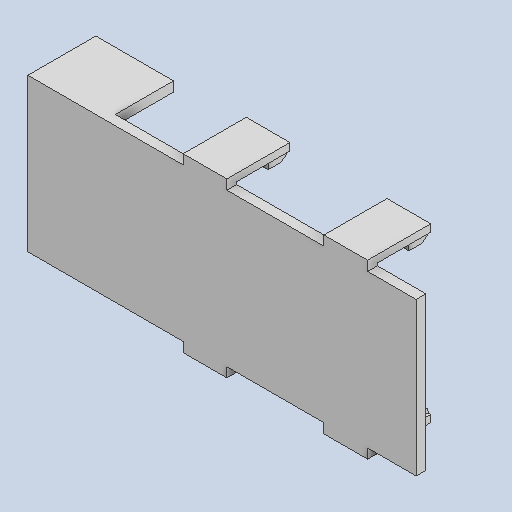
# Autodesk Inventor part: np2_cap_open_top
Saved by Autodesk Inventor 2025 (Build 290162000, 162)
## iProperties
Created: 2023-11-21
Part Number: np2_cap_open_top
Material: Generic
Document SubType Name: Modeling
Designer: mmelin
Density: 1 g/cm^3
Appearance: Default
Author: mmelin
Autodesk Inventor part; units mm, degrees
ref_plane "YZ Plane" through (0, 0, 0) normal (1, 0, 0) x (0, 1, 0)
ref_plane "XZ Plane" through (0, 0, 0) normal (0, 1, 0) x (-1, 0, 0)
sketch "Sketch1" plane through (0, 0, 0) normal (0, 0, 1) x (1, 0, 0)
  line L0 (1, -0.6) -> (1, -5.45) projected
  line L1 (-15, 0) -> (-11.6, 0)
  line L2 (-6.8, -6.3) -> (-8.6, -6.3) projected
  line L3 (-8.6, 0) -> (-6.8, 0) projected
  line L4 (-2.8, 0) -> (-1, 0) projected
  line L5 (-6.8, -6.3) -> (-8.6, -6.3) projected
  line L6 (-1, -6.3) -> (-2.8, -6.3) projected
  line L7 (-8.6, -6.3) -> (-6.8, -6.3)
  line L8 (-6.8, -6.3) -> (-6.8, -6.7)
  line L9 (-6.8, -6.7) -> (-8.6, -6.7)
  line L10 (-8.6, -6.7) -> (-8.6, -6.3)
  line L11 (-8.6, 0) -> (-6.8, 0)
  line L12 (-6.8, 0) -> (-6.8, 0.4)
  line L13 (-6.8, 0.4) -> (-8.6, 0.4)
  line L14 (-8.6, 0.4) -> (-8.6, 0)
  line L15 (-2.8, 0) -> (-1, 0)
  line L16 (-1, 0) -> (-1, 0.4)
  line L17 (-1, 0.4) -> (-2.8, 0.4)
  line L18 (-2.8, 0.4) -> (-2.8, 0)
  line L19 (-2.8, -6.3) -> (-1, -6.3)
  line L20 (-1, -6.3) -> (-1, -6.7)
  line L21 (-1, -6.7) -> (-2.8, -6.7)
  line L22 (-2.8, -6.7) -> (-2.8, -6.3)
  line L23 (-8.6, -5.9) -> (-8.6, -6.3) projected
  line L24 (-6.8, -5.9) -> (-6.8, -6.3) projected
  line L25 (-2.8, -5.9) -> (-2.8, -6.3) projected
  line L26 (-1, -5.9) -> (-1, -6.3) projected
  line L27 (1, -6.3) -> (-15, -6.3)
  line L28 (-15, -6.3) -> (-15, 0)
  line L29 (-15, 0) -> (1, 0)
  line L30 (1, 0) -> (1, -6.3)
  line L31 (-15, -1.7791) -> (-15, -4.5209) projected
  point P0 (0, 0)
  dimension "d2" = 0.4
  constraints: 42 end point, 16 collinear, 10 parallel, 5 horizontal, 5 perpendicular, 3 equal length
  measures "d2" distance of L7.end L8.end
extrude "Extrusion1" add sketch "Sketch1" along normal blind 0.4
sketch "Sketch2" plane through (0, 0, 0) normal (0, 0, -1) x (-1, 0, 0)
  line L0 (8.6, -6.7) -> (6.8, -6.7) projected
  line L1 (6.8, -6.7) -> (6.8, -6.3) projected
  line L2 (8.6, -6.7) -> (6.8, -6.7)
  line L3 (6.8, -6.7) -> (6.8, -6.4)
  line L4 (6.8, -6.4) -> (8.6, -6.4)
  line L5 (8.6, -6.4) -> (8.6, -6.7)
  line L6 (2.8, -6.3) -> (2.8, -6.7) projected
  line L7 (1, -6.7) -> (1, -6.3) projected
  line L8 (2.8, -6.7) -> (1, -6.7)
  line L9 (1, -6.7) -> (1, -6.4)
  line L10 (1, -6.4) -> (2.8, -6.4)
  line L11 (2.8, -6.4) -> (2.8, -6.7)
  line L12 (1, 0) -> (1, 0.4) projected
  line L13 (2.8, 0.4) -> (2.8, 0) projected
  line L14 (1, 0.4) -> (2.8, 0.4)
  line L15 (2.8, 0.4) -> (2.8, 0.1)
  line L16 (2.8, 0.1) -> (1, 0.1)
  line L17 (1, 0.1) -> (1, 0.4)
  line L18 (6.8, 0.4) -> (8.6, 0.4) projected
  line L19 (8.6, 0.4) -> (8.6, 0) projected
  line L20 (6.8, 0.4) -> (8.6, 0.4)
  line L21 (8.6, 0.4) -> (8.6, 0.1)
  line L22 (8.6, 0.1) -> (6.8, 0.1)
  line L23 (6.8, 0.1) -> (6.8, 0.4)
  line L24 (6.8, -6.3) -> (2.8, -6.3) projected
  line L25 (2.8, 0) -> (6.8, 0) projected
  point P0 (0, 0)
  dimension "d3" = 0.1
  dimension "d4" = 0.1
  constraints: 32 end point, 8 parallel, 4 horizontal, 4 perpendicular, 4 point on line, 2 collinear
  measures "d3" distance between parallel lines of L4 L24
  measures "d4" distance between parallel lines of L25 L22
ref_plane "Work Plane1" through (-8.6, -0.4, -2.2) normal (0, 0, 1) x (1, 0, 0)
extrude "Extrusion2" add sketch "Sketch2" along normal up to surface (2.2 mm away)
sketch "Sketch3" plane through (-8.6, 0.1, 0) normal (0, -1, 0) x (1, 0, 0)
  line L0 (0.1, -1.4) -> (1.7, -1.4)
  line L1 (1.7, -1.4) -> (1.7, -2.2)
  line L2 (1.7, -2.2) -> (0.1, -2.2)
  line L3 (0.1, -2.2) -> (0.1, -1.4)
  line L4 (5.9, -1.4) -> (7.5, -1.4)
  line L5 (7.5, -1.4) -> (7.5, -2.2)
  line L6 (7.5, -2.2) -> (5.9, -2.2)
  line L7 (5.9, -2.2) -> (5.9, -1.4)
  line L8 (1.8, -2.2) -> (1.8, -1.2) projected
  line L9 (1.8, -1.2) -> (0, -1.2) projected
  line L10 (0, -2.2) -> (1.8, -2.2) projected
  line L11 (0, -1.2) -> (0, -2.2) projected
  line L12 (7.6, -2.2) -> (7.6, -1.2) projected
  line L13 (5.8, -2.2) -> (7.6, -2.2) projected
  line L14 (7.6, -1.2) -> (5.8, -1.2) projected
  line L15 (5.8, -1.2) -> (5.8, -2.2) projected
  line L16 (1.8, -2.2) -> (0, -2.2) projected
  line L17 (7.6, -2.2) -> (5.8, -2.2) projected
  point P0 (8.6, 0)
  point P1 (6.7, -1.2)
  dimension "d7" = 0.1
  dimension "d8" = 0.2
  dimension "d9" = 0.1
  dimension "d10" = 0.1
  dimension "d11" = 0.2
  dimension "d12" = 0.1
  constraints: 16 end point, 4 parallel, 2 collinear, 2 horizontal, 2 perpendicular, 1 midpoint
  measures "d7" distance between parallel lines of L11 L3
  measures "d8" distance between parallel lines of L9 L0
  measures "d9" distance between parallel lines of L8 L1
  measures "d10" distance between parallel lines of L15 L7
  measures "d11" distance from line of point (6.7, -1.2) L4
  measures "d12" distance between parallel lines of L12 L5
extrude "Extrusion3" add sketch "Sketch3" along normal blind 0.35 draft -5 contours L0 L1 L2 L3 | L4 L5 L6 L7
sketch "Sketch4" plane through (-2.8, -6.4, 0) normal (0, 1, 0) x (1, 0, 0)
  line L0 (-4.1, 2.2) -> (-5.7, 2.2) projected
  line L1 (-5.7, 2.2) -> (-5.7, 1.4) projected
  line L2 (-4.1, 1.4) -> (-4.1, 2.2) projected
  line L3 (-5.7, 1.4) -> (-4.1, 1.4) projected
  line L4 (0.1, 1.4) -> (1.7, 1.4) projected
  line L5 (0.1, 2.2) -> (0.1, 1.4) projected
  line L6 (1.7, 2.2) -> (0.1, 2.2) projected
  line L7 (1.7, 1.4) -> (1.7, 2.2) projected
  point P0 (2.8, 0)
extrude "Extrusion4" add sketch "Sketch4" along normal blind 0.35 draft -5
chamfer "Chamfer1" distance 0.2 angle 45 4 edges at (-1.9, -0.25, -2.1694) (-7.7, -0.25, -2.1694) (-1.9, -6.05, -2.1694) (-7.7, -6.05, -2.1694)
sketch "Sketch5" plane through (0, 0, 0) normal (0, 0, -1) x (-1, 0, 0)
  line L0 (15, -6.3) -> (11.8, -6.3)
  line L1 (11.8, -6.3) -> (11.8, -5.9)
  line L2 (11.8, -5.9) -> (15, -5.9)
  line L3 (15, -5.9) -> (15, -6.3)
  line L4 (8.6, 0) -> (15, 0) projected
  line L5 (15, 0) -> (11.8, 0)
  line L6 (11.8, 0) -> (11.8, -0.4)
  line L7 (11.8, -0.4) -> (15, -0.4)
  line L8 (15, -0.4) -> (15, 0)
  line L9 (11.6, 0) -> (11.6, -0.4) projected
  line L10 (11.6, -5.9) -> (11.6, -6.3) projected
  point P0 (0, 0)
  dimension "d20" = 0.2
  dimension "d21" = 0.2
  constraints: 16 end point, 6 parallel, 2 horizontal, 2 perpendicular
  measures "d20" distance between parallel lines of L6 L9
  measures "d21" distance between parallel lines of L10 L1
extrude "Extrusion5" add sketch "Sketch5" along normal blind 2.4
sketch "Sketch6" plane through (0, 0, 0) normal (0, 0, -1) x (-1, 0, 0)
  line L0 (15, -0.4) -> (15, -5.9) projected
  line L1 (15, -5.9) -> (14.7, -5.9)
  line L2 (14.7, -5.9) -> (14.7, -0.4)
  line L3 (14.7, -0.4) -> (15, -0.4)
  line L4 (15, -0.4) -> (15, -5.9)
  line L5 (15, -0.4) -> (11.8, -0.4) projected
  point P0 (0, 0)
  dimension "d24" = 0.3
  constraints: 8 end point, 2 parallel, 1 collinear, 1 horizontal, 1 perpendicular
  measures "d24" distance between parallel lines of L4 L2
extrude "Extrusion6" add sketch "Sketch6" along normal blind 2.1
equation "\"d8\" = d11"
equation "\"d9\" = d7"
equation "\"d10\" = d7"
equation "\"d12\" = d7"
equation "\"d21\" = d20"
body "Solid1"
